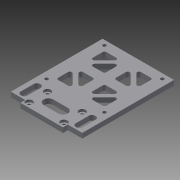
# Autodesk Inventor part: nuccase_hold
Saved by Autodesk Inventor 2015 (Build 190159000, 159)
## iProperties
Created: 2016-10-24
Part Number: nuccase_hold
Material: Generic
Document SubType Name: Modeling
Designer: Bardo91
Density: 1 g/cm^3
Appearance: Default
Author: Bardo91
Autodesk Inventor part; units mm, degrees
ref_plane "YZ Plane" through (0, 0, 0) normal (1, 0, 0) x (0, 1, 0)
ref_plane "XZ Plane" through (0, 0, 0) normal (0, 1, 0) x (-1, 0, 0)
ref_plane "XY Plane" through (0, 0, 0) normal (0, 0, 1) x (1, 0, 0)
sketch "Sketch1" plane through (0, 0, 0) normal (0, 0, 1) x (1, 0, 0)
  line L0 (0, 0) -> (36, 0)
  line L1 (36, 0) -> (36, 19)
  line L2 (36, 19) -> (0, 19)
  circle A0 centre (0, 19) radius 1.75
  circle A1 centre (0, 0) radius 1.75
  circle A2 centre (36, 0) radius 1.75
  circle A3 centre (36, 19) radius 1.75
  line L3 (0, 0) -> (0, -5)
  line L4 (0, -5) -> (40, -5)
  line L5 (0, -5) -> (-4, -5)
  line L6 (-4, -5) -> (-4, 25)
  line L7 (-4, 25) -> (40, 25)
  line L8 (40, 25) -> (40, -5)
  line L9 (36, 0) -> (36, 30)
  line L10 (36, 30) -> (0, 30)
  line L11 (18, 30) -> (48, 30)
  line L12 (48, 30) -> (48, 90)
  line L13 (48, 90) -> (-12, 90)
  line L14 (-12, 90) -> (-12, 30)
  line L15 (-4, 0) -> (-19, 0)
  line L16 (-19, 0) -> (-19, 95)
  line L17 (40, 0) -> (55, 0)
  line L18 (55, 0) -> (55, 95)
  line L19 (55, 95) -> (-19, 95)
  circle A4 centre (-12, 90) radius 1.75
  circle A5 centre (48, 90) radius 1.75
  circle A6 centre (-12, 30) radius 1.75
  circle A7 centre (48, 30) radius 1.75
  dimension "d0" = 36
  dimension "d1" = 19
  dimension "d2" = 3.5
  dimension "d3" = 3.5
  dimension "d4" = 3.5
  dimension "d5" = 3.5
  dimension "d6" = 5
  dimension "d7" = 40
  dimension "d8" = 4
  dimension "d9" = 30
  dimension "d10" = 30
  dimension "d11" = 30
  dimension "d12" = 60
  dimension "d13" = 60
  dimension "d14" = 15
  dimension "d15" = 95
  dimension "d16" = 15
  dimension "d17" = 3.5
  dimension "d18" = 3.5
  dimension "d19" = 3.5
  dimension "d20" = 3.5
  constraints: 40 end point, 14 perpendicular, 8 centre point, 8 coincident, 5 point on line, 3 horizontal, 1 midpoint, 1 vertical
  measures "d0" distance of L0.start L0.end
  measures "d1" distance of L0.end L1.end
  measures "d2" diameter of A0
  measures "d3" diameter of A1
  measures "d4" diameter of A2
  measures "d5" diameter of A3
  measures "d6" distance of L3.start L3.end
  measures "d7" distance of L3.end L4.end
  measures "d8" distance of L3.end L5.end
  measures "d9" distance of L5.end L6.end
  measures "d10" distance of L9.start L9.end
  measures "d11" distance of L11.start L11.end
  measures "d12" distance of L11.end L12.end
  measures "d13" distance of L12.end L13.end
  measures "d14" distance of L15.start L15.end
  measures "d15" distance of L15.end L16.end
  measures "d16" distance of L17.start L17.end
  measures "d17" diameter of A4
  measures "d18" diameter of A5
  measures "d19" diameter of A6
  measures "d20" diameter of A7
extrude "Extrusion1" add sketch "Sketch1" along normal blind 5 contours A1 L3 L5 L6 L7 L9 A3 L1 A2 L0 | L0 A2 L1 A3 L9 L7 L8 L4 L3 A1 | L8 L7 L6 L15 L16 L19 L18 L17
sketch "Sketch2" plane through (0, 0, 5) normal (0, 0, 1) x (1, 0, 0)
  circle A0 centre (0, 19) radius 1.75 projected
  circle A1 centre (0, 19) radius 3.5
  circle A2 centre (0, 0) radius 3.5
  circle A3 centre (36, 0) radius 1.75 projected
  circle A4 centre (36, 0) radius 3.5
  circle A5 centre (36, 19) radius 3.5
  dimension "d23" = 7
  dimension "d24" = 7
  dimension "d25" = 7
  dimension "d26" = 7
  constraints: 4 centre point, 3 coincident
  measures "d23" diameter of A1
  measures "d24" diameter of A2
  measures "d25" diameter of A4
  measures "d26" diameter of A5
extrude "Extrusion2" cut sketch "Sketch2" against normal blind 2.5
sketch "Sketch3" plane through (0, 0, 0) normal (0, 0, -1) x (-1, 0, 0)
  circle A0 centre (-48, 30) radius 1.75 projected
  circle A1 centre (-48, 30) radius 3.5
  circle A2 centre (-48, 90) radius 1.75 projected
  circle A3 centre (-48, 90) radius 3.5
  circle A4 centre (12, 90) radius 1.75 projected
  circle A5 centre (12, 90) radius 3.5
  circle A6 centre (12, 30) radius 1.75 projected
  circle A7 centre (12, 30) radius 3.5
  point P0 (0, 0)
  dimension "d29" = 7
  dimension "d30" = 7
  dimension "d31" = 7
  dimension "d32" = 7
  constraints: 4 centre point, 4 coincident
  measures "d29" diameter of A1
  measures "d30" diameter of A3
  measures "d31" diameter of A5
  measures "d32" diameter of A7
extrude "Extrusion3" cut sketch "Sketch3" against normal blind 2.5
sketch "Sketch5" plane through (0, 0, 5) normal (0, 0, 1) x (1, 0, 0)
  circle A0 centre (0, 0) radius 1.75 projected
  line L0 (0, 0) -> (0, 5)
  line L1 (0, 5) -> (5, 5)
  line L2 (5, 10) -> (5, 10)
  line L3 (10, 15) -> (25, 15)
  line L4 (30, 10) -> (30, 10)
  line L5 (25, 5) -> (10, 5)
  arc A1 (10, 15) -> (5, 10) centre (10, 10) ccw
  arc A2 (5, 10) -> (10, 5) centre (10, 10) ccw
  arc A3 (30, 10) -> (25, 15) centre (25, 10) ccw
  arc A4 (25, 5) -> (30, 10) centre (25, 10) ccw
  line L6 (-19, 0) -> (-14, 0)
  line L7 (-19, 0) -> (-4, 0) projected
  line L8 (-14, 0) -> (-14, 2)
  line L9 (-11, 2) -> (-10, 2)
  line L10 (-7, 5) -> (-7, 19)
  line L11 (-10, 22) -> (-11, 22)
  line L12 (-14, 19) -> (-14, 5)
  line L13 (-4, -5) -> (40, -5) projected
  line L14 (18, -5) -> (18, 1)
  arc A5 (-11, 22) -> (-14, 19) centre (-11, 19) ccw
  arc A6 (-7, 19) -> (-10, 22) centre (-10, 19) ccw
  arc A7 (-10, 2) -> (-7, 5) centre (-10, 5) ccw
  arc A8 (-14, 5) -> (-11, 2) centre (-11, 5) ccw
  line L15 (47, 2) -> (46, 2)
  line L16 (43, 5) -> (43, 19)
  line L17 (46, 22) -> (47, 22)
  line L18 (50, 19) -> (50, 5)
  arc A9 (50, 19) -> (47, 22) centre (47, 19) ccw
  arc A10 (46, 22) -> (43, 19) centre (46, 19) ccw
  arc A11 (43, 5) -> (46, 2) centre (46, 5) ccw
  arc A12 (47, 2) -> (50, 5) centre (47, 5) ccw
  line L19 (18, 0) -> (18, 95)
  line L20 (55, 95) -> (-19, 95) projected
  circle A13 centre (-12, 30) radius 1.75 projected
  circle A14 centre (-12, 90) radius 1.75 projected
  line L21 (-12, 30) -> (-12, 90)
  line L22 (-12, 60) -> (18, 60)
  line L23 (-12, 90) -> (18, 90)
  circle A15 centre (-12, 90) radius 3.5 projected
  line L24 (-12, 90) -> (-7, 90)
  line L25 (-7, 90) -> (-7, 85)
  line L26 (-5, 85) -> (5.1716, 85)
  line L27 (-7, 83) -> (-7, 72.8284)
  line L28 (-3.5858, 71.4142) -> (6.5858, 81.5858)
  line L29 (18, 60) -> (18, 65)
  line L30 (18, 65) -> (13, 65)
  line L31 (11, 65) -> (0.8284, 65)
  line L32 (13, 67) -> (13, 77.1716)
  line L33 (9.5858, 78.5858) -> (-0.5858, 68.4142)
  arc A16 (6.5858, 81.5858) -> (5.1716, 85) centre (5.1716, 83) ccw
  arc A17 (-5, 85) -> (-7, 83) centre (-5, 83) ccw
  arc A18 (-7, 72.8284) -> (-3.5858, 71.4142) centre (-5, 72.8284) ccw
  arc A19 (-0.5858, 68.4142) -> (0.8284, 65) centre (0.8284, 67) ccw
  arc A20 (13, 77.1716) -> (9.5858, 78.5858) centre (11, 77.1716) ccw
  arc A21 (11, 65) -> (13, 67) centre (11, 67) ccw
  circle A22 centre (-12, 30) radius 3.5
  line L34 (-5, 35) -> (5.1716, 35)
  line L35 (-7, 37) -> (-7, 47.1716)
  line L36 (-3.5858, 48.5858) -> (6.5858, 38.4142)
  line L37 (11, 55) -> (0.8284, 55)
  line L38 (13, 53) -> (13, 42.8284)
  line L39 (9.5858, 41.4142) -> (-0.5858, 51.5858)
  arc A23 (5.1716, 35) -> (6.5858, 38.4142) centre (5.1716, 37) ccw
  arc A24 (-7, 37) -> (-5, 35) centre (-5, 37) ccw
  arc A25 (-3.5858, 48.5858) -> (-7, 47.1716) centre (-5, 47.1716) ccw
  arc A26 (0.8284, 55) -> (-0.5858, 51.5858) centre (0.8284, 53) ccw
  arc A27 (9.5858, 41.4142) -> (13, 42.8284) centre (11, 42.8284) ccw
  arc A28 (13, 53) -> (11, 55) centre (11, 53) ccw
  line L40 (41, 85) -> (30.8284, 85)
  line L41 (43, 83) -> (43, 72.8284)
  line L42 (39.5858, 71.4142) -> (29.4142, 81.5858)
  line L43 (25, 65) -> (35.1716, 65)
  line L44 (23, 67) -> (23, 77.1716)
  line L45 (26.4142, 78.5858) -> (36.5858, 68.4142)
  arc A29 (30.8284, 85) -> (29.4142, 81.5858) centre (30.8284, 83) ccw
  arc A30 (43, 83) -> (41, 85) centre (41, 83) ccw
  arc A31 (39.5858, 71.4142) -> (43, 72.8284) centre (41, 72.8284) ccw
  arc A32 (35.1716, 65) -> (36.5858, 68.4142) centre (35.1716, 67) ccw
  arc A33 (26.4142, 78.5858) -> (23, 77.1716) centre (25, 77.1716) ccw
  arc A34 (23, 67) -> (25, 65) centre (25, 67) ccw
  line L46 (43, 37) -> (43, 47.1716)
  arc A35 (41, 35) -> (43, 37) centre (41, 37) ccw
  arc A36 (43, 47.1716) -> (39.5858, 48.5858) centre (41, 47.1716) ccw
  line L47 (39.5858, 48.5858) -> (29.4142, 38.4142)
  line L48 (26.4142, 41.4142) -> (36.5858, 51.5858)
  line L49 (25, 55) -> (35.1716, 55)
  line L50 (23, 53) -> (23, 42.8284)
  line L51 (41, 35) -> (30.8284, 35)
  arc A37 (29.4142, 38.4142) -> (30.8284, 35) centre (30.8284, 37) ccw
  arc A38 (23, 42.8284) -> (26.4142, 41.4142) centre (25, 42.8284) ccw
  arc A39 (36.5858, 51.5858) -> (35.1716, 55) centre (35.1716, 53) ccw
  arc A40 (25, 55) -> (23, 53) centre (25, 53) ccw
  point P0 (5, 15)
  point P1 (30, 15)
  point P2 (30, 5)
  point P3 (-7, 2)
  point P4 (-7, 22)
  point P5 (-14, 22)
  point P6 (50, 2)
  point P7 (43, 2)
  point P8 (43, 22)
  point P9 (50, 22)
  point P10 (10, 85)
  point P11 (-7, 68)
  point P12 (-4, 65)
  point P13 (13, 82)
  point P14 (-7, 35)
  point P15 (10, 35)
  point P16 (-7, 52)
  point P17 (13, 55)
  point P18 (-4, 55)
  point P19 (13, 38)
  point P20 (43, 85)
  point P21 (26, 85)
  point P22 (43, 68)
  point P23 (23, 65)
  point P24 (40, 65)
  point P25 (23, 82)
  point P26 (26, 35)
  point P27 (23, 38)
  point P28 (43, 52)
  point P29 (40, 55)
  point P30 (43, 35)
  point P31 (23, 55)
  dimension "d40" = 5
  dimension "d41" = 5
  dimension "d42" = 10
  dimension "d43" = 25
  dimension "d44" = 5
  dimension "d45" = 5
  dimension "d46" = 2
  dimension "d47" = 7
  dimension "d48" = 20
  dimension "d49" = 3
  dimension "d50" = 5
  dimension "d51" = 5
  dimension "d52" = 17
  dimension "d53" = 17
  dimension "d54" = 5
  dimension "d55" = 5
  dimension "d56" = 17
  dimension "d57" = 17
  dimension "d58" = 2
  constraints: 98 end point, 89 symmetric about line, 77 point on line, 72 point on circle, 37 centre point, 28 tangent, 15 perpendicular, 11 equal radius, 5 vertical, 3 midpoint, 23 other
  measures "d40" distance of L0.start L0.end
  measures "d41" distance of L0.end L1.end
  measures "d42" distance of L1.end point (5, 15)
  measures "d43" distance of point (5, 15) point (30, 15)
  measures "d44" radius of A1
  measures "d45" distance of L6.start L6.end
  measures "d46" distance of L6.end L8.end
  measures "d47" distance of L8.end point (-7, 2)
  measures "d48" distance of point (-7, 2) point (-7, 22)
  measures "d49" radius of A5
  measures "d50" distance of L24.start L24.end
  measures "d51" distance of L24.end L25.end
  measures "d52" distance of L25.end point (10, 85)
  measures "d53" distance of L25.end point (-7, 68)
  measures "d54" distance of L22.end L29.end
  measures "d55" distance of L29.end L30.end
  measures "d56" distance of L30.end point (-4, 65)
  measures "d57" distance of L30.end point (13, 82)
  measures "d58" radius of A16
extrude "Extrusion5" cut sketch "Sketch5" against normal through all contours L3 L19 L5 A2 A1 | L3 A3 A4 L5 L19 | A8 L12 A5 L11 A6 L10 A7 L9 | L15 A11 L16 A10 L17 A9 L18 A12 | L26 A16 L28 A18 L27 A17 | L31 A19 L33 A20 L32 A21 | A24 L35 A25 L36 A23 L34 | A28 L38 A27 L39 A26 L37 | A30 L41 A31 L42 A29 L40 | A34 L44 A33 L45 A32 L43 | A35 L51 A37 L47 A36 L46 | A38 L50 A40 L49 A39 L48
body "Solid1"
